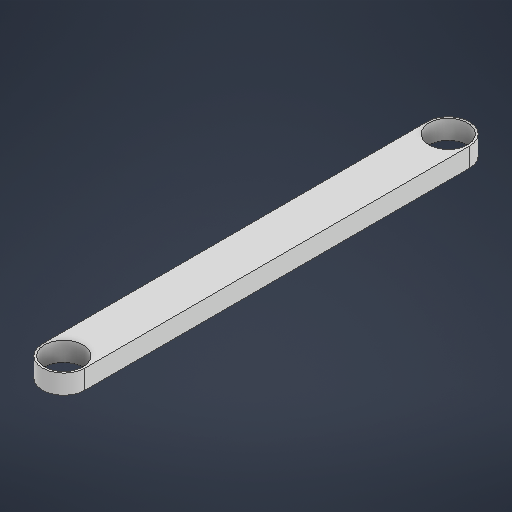
# Autodesk Inventor part: tibia
Saved by Autodesk Inventor 2027 (Build 310192060, 192F)
## iProperties
Created: 2026-08-02
Part Number: tibia
Material: Ogólny
Document SubType Name: Modeling
Designer: User
Density: 1 g/cm^3
Appearance: Domyślna
Author: User
Autodesk Inventor part; units mm, degrees
ref_plane "YZ Plane" through (0, 0, 0) normal (1, 0, 0) x (0, 1, 0)
ref_plane "XZ Plane" through (0, 0, 0) normal (0, 1, 0) x (-1, 0, 0)
ref_plane "XY Plane" through (0, 0, 0) normal (0, 0, 1) x (1, 0, 0)
sketch "Szkic1" plane through (0, 0, 0) normal (0, 1, 0) x (-1, 0, 0)
  line L0 (0, 0) -> (0, -20) construction
  line L1 (-1.1, 0) -> (-1.1, -20)
  line L2 (1.1, -20) -> (1.1, 0)
  arc A0 (1.1, 0) -> (-1.1, 0) centre (0, 0) ccw
  arc A1 (-1.1, -20) -> (1.1, -20) centre (0, -20) ccw
  circle A2 centre (0, 0) radius 1
  circle A3 centre (0, -20) radius 1
  point P0 (0, -10)
  dimension "d0" = 20
  dimension "d1" = 2.2
  dimension "d2" = 2
  dimension "d3" = 2
  constraints: 8 end point, 4 centre point, 4 point on circle, 4 tangent, 2 coincident, 1 midpoint, 1 parallel, 1 vertical
  measures "d0" distance of L0.start L0.end
  measures "d1" diameter of A1
  measures "d2" diameter of A2
  measures "d3" diameter of A3
extrude "Wyciągnięcie proste1" add sketch "Szkic1" along normal blind 1
